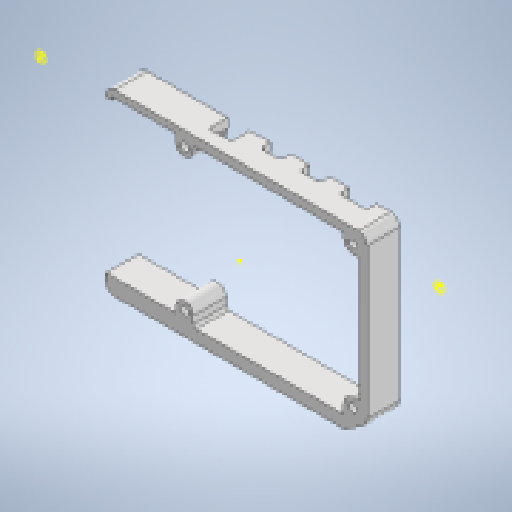
# Autodesk Inventor part: rpi_wspornik
Saved by Autodesk Inventor 2023.4 (Build 274418000, 418)
## iProperties
Created: 2024-09-15
Part Number: rpi_wspornik
Material: Generic
Document SubType Name: Modeling
Designer: komputer
Density: 1 g/cm^3
Appearance: Default
Author: komputer
Autodesk Inventor part; units mm, degrees
ref_plane "YZ Plane" through (0, 0, 0) normal (1, 0, 0) x (0, 1, 0)
ref_plane "XZ Plane" through (0, 0, 0) normal (0, 1, 0) x (-1, 0, 0)
ref_plane "XY Plane" through (0, 0, 0) normal (0, 0, 1) x (1, 0, 0)
sketch "Sketch1" plane through (0, 0, 0) normal (0, 0, 1) x (1, 0, 0)
  circle A0 centre (39, 24.5) radius 1.35 projected
  circle A1 centre (-19, 24.5) radius 1.35 projected
  circle A2 centre (-19, -24.5) radius 1.35 projected
  circle A3 centre (39, -24.5) radius 1.35 projected
  arc A4 (42.9875, 27.416) -> (40.9875, 29.416) centre (40.9875, 27.416) ccw projected
  line L0 (42.9875, 27.416) -> (42.9875, -26.5136) projected
  line L1 (-21.0125, 29.416) -> (40.9875, 29.416) projected
  arc A5 (42.0969, -28.1777) -> (42.9875, -26.5136) centre (40.9875, -26.5136) ccw projected
  line L2 (42.0969, -28.1777) -> (31.1281, -35.4903) projected
  line L3 (-29.6767, -31.7482) -> (-23.5983, -25.6698) projected
  line L4 (-23.5983, -25.6698) -> (-23.0125, -24.2556) projected
  line L5 (-23.0125, -24.2556) -> (-23.0125, 27.416) projected
  arc A6 (-21.0125, 29.416) -> (-23.0125, 27.416) centre (-21.0125, 27.416) ccw projected
  line L6 (-42.5, 25) -> (-42.5, -25) projected
  circle A7 centre (39, 24.5) radius 3
  circle A8 centre (-19, 24.5) radius 3
  circle A9 centre (39, -24.5) radius 3
  circle A10 centre (-19, -24.5) radius 3
  line L7 (36, -21.5) -> (42, -21.5)
  line L8 (42, -21.5) -> (42, -27.5)
  line L9 (42, -27.5) -> (36, -27.5)
  line L10 (36, -27.5) -> (36, -21.5)
  line L11 (36, -21.5) -> (42, -27.5) construction
  line L12 (42, -21.5) -> (36, -27.5) construction
  line L13 (36, -27.5) -> (36, -32.2423)
  line L14 (42, -21.5) -> (42.9875, -21.5)
  line L15 (42.5, -25) -> (42.5, 25) projected
  line L16 (41.5, -21.5) -> (41.5, 38.929)
  line L17 (40, 10.3) -> (39.15, 10.3) projected
  line L18 (42.9875, 11.3) -> (36.4675, 11.3)
  line L19 (40.35, 24.5) -> (42.9875, 24.5)
  line L20 (46.88, 26.416) -> (-24.7177, 26.416)
  line L21 (-16, 24.5) -> (-16, 26.416)
  line L22 (-22, 24.5) -> (-22, 26.416)
  line L23 (-22, 26.416) -> (-22, 29.1552)
  point P0 (0, 0)
  point P1 (36.6915, 26.416)
  point P2 (41.3085, 26.416)
  point P3 (41.5, 26.416)
  point P4 (41.5, 26.1583)
  point P5 (41.5, 22.8417)
  point P6 (41.5, 24.5)
  point P7 (42.5, 24.5)
  point P8 (42.5, 11.3)
  point P9 (41.5, 11.3)
  point P10 (39, -21.5)
  point P11 (36, -24.5)
  dimension "d0" = 6
  dimension "d1" = 6
  dimension "d2" = 6
  dimension "d3" = 6
  dimension "d4" = 1
  dimension "d5" = 1
  dimension "d6" = 3
  constraints: 30 end point, 8 point on line, 5 perpendicular, 4 centre point, 4 coincident, 3 horizontal, 3 parallel, 3 point on circle, 2 midpoint, 1 horizontal alignment, 1 vertical, 1 other
  measures "d0" diameter of A7
  measures "d1" diameter of A8
  measures "d2" diameter of A9
  measures "d3" diameter of A10
  measures "d4" distance between parallel lines of L15 L16
  measures "d5" distance between parallel lines of L18 L17
  measures "d6" distance between parallel lines of L1 L20
extrude "Extrusion1" add sketch "Sketch1" along normal blind 11.2 contours L0 L20 L16 A4 | L16 L20 A7 A8 L23 A6 L1 A4 | L0 L19 A7 L16 L20 | L16 A7 L20 | L0 L18 L15 L19 | L16 A7 L20 | A7 L19 L16 | L20 A7 | L0 L14 L15 L18 | L0 A5 L2 L13 L9 L8 L14 | L15 L14 L7 L16 L18 | L20 A8 L22 | L21 A8 L20 | L20 A8 | A8 L20 | L8 A9 L7 | A9 | L8 L9 A9 | L10 A9 L9 | A10 picked at (41.5914, 25.4334)
sketch "Sketch2" plane through (0, 0, 11.2) normal (0, 0, 1) x (1, 0, 0)
  line L0 (-39.5, -28) -> (39.5, -28) projected
  line L1 (36, -32.2423) -> (42.0969, -28.1777) projected
  circle A0 centre (-19, -24.5) radius 3 projected
  line L2 (36, -32.2423) -> (-22, -32.2423)
  line L3 (-22, -32.2423) -> (-22, -24.5)
  line L4 (-16, -24.5) -> (-16, -28)
  line L5 (36, -24.5) -> (36, -32.2423) projected
  point P0 (0, 0)
  point P1 (36, -28)
  constraints: 6 end point, 2 perpendicular, 2 point on circle, 1 horizontal, 1 point on line, 1 tangent
extrude "Extrusion2" add sketch "Sketch2" against normal up to surface (11.2 mm away) contours L3 A0 L4 L0 | L0 L5 L2 L3
sketch "Sketch3" plane through (0, 0, 0) normal (0, 0, -1) x (-1, 0, 0)
  line L0 (-35.77, 29.5) -> (-35.77, 28.6) projected
  line L1 (-26.83, 29.5) -> (-26.83, 28.6) projected
  line L2 (-19.75, 28.35) -> (-19.75, 29.8) projected
  line L3 (-13.25, 29.8) -> (-13.25, 28.35) projected
  line L4 (-6.25, 28.35) -> (-6.25, 29.8) projected
  line L5 (0.25, 29.8) -> (0.25, 28.35) projected
  line L6 (8, 24.9) -> (8, 27) projected
  line L7 (15, 27) -> (15, 24.9) projected
  line L8 (-35.77, 29.5) -> (-26.83, 29.5)
  line L9 (-26.83, 29.5) -> (-26.83, 26.142)
  line L10 (-26.83, 26.142) -> (-35.77, 26.142)
  line L11 (-35.77, 26.142) -> (-35.77, 29.5)
  line L12 (-19.75, 29.8) -> (-13.15, 29.8)
  line L13 (-13.15, 29.8) -> (-13.15, 26.142)
  line L14 (-13.15, 26.142) -> (-19.75, 26.142)
  line L15 (-19.75, 26.142) -> (-19.75, 29.8)
  line L16 (-6.25, 29.8) -> (0.35, 29.8)
  line L17 (0.35, 29.8) -> (0.35, 26.142)
  line L18 (0.35, 26.142) -> (-6.25, 26.142)
  line L19 (-6.25, 26.142) -> (-6.25, 29.8)
  line L20 (-26.53, 25.842) -> (-26.53, 29.8)
  line L21 (-26.53, 29.8) -> (-36.07, 29.8)
  line L22 (-36.07, 29.8) -> (-36.07, 25.842)
  line L23 (-36.07, 25.842) -> (-26.53, 25.842)
  line L24 (-20.05, 25.842) -> (-12.85, 25.842)
  line L25 (-12.85, 25.842) -> (-12.85, 30.1)
  line L26 (-12.85, 30.1) -> (-20.05, 30.1)
  line L27 (-20.05, 30.1) -> (-20.05, 25.842)
  line L28 (-6.55, 25.842) -> (0.65, 25.842)
  line L29 (0.65, 25.842) -> (0.65, 30.1)
  line L30 (0.65, 30.1) -> (-6.55, 30.1)
  line L31 (-6.55, 30.1) -> (-6.55, 25.842)
  line L32 (8, 30.3074) -> (15, 30.3074)
  line L33 (15, 30.3074) -> (15, 24.9)
  line L34 (15, 24.9) -> (8, 24.9)
  line L35 (8, 24.9) -> (8, 30.3074)
  line L36 (7.7, 24.6) -> (15.3, 24.6)
  line L37 (15.3, 24.6) -> (15.3, 30.6074)
  line L38 (15.3, 30.6074) -> (7.7, 30.6074)
  line L39 (7.7, 30.6074) -> (7.7, 24.6)
  line L40 (2.5, 26.8) -> (2.5, 23.7709) projected
  line L41 (5.5, 26.8) -> (5.5, 23.7709) projected
  line L42 (5.5, 23.7709) -> (2.5, 23.7709)
  line L43 (2.5, 23.7709) -> (2.5, 28.416)
  line L44 (2.5, 28.416) -> (5.5, 28.416)
  line L45 (5.5, 28.416) -> (5.5, 23.7709)
  line L46 (-40.9875, 29.416) -> (21.0125, 29.416) projected
  point P0 (0, 0)
  dimension "d11" = 0.3
  dimension "d12" = 0.3
  dimension "d13" = 0.3
  dimension "d14" = 0.3
  dimension "d15" = 1
  constraints: 72 end point, 18 parallel, 9 perpendicular, 5 horizontal, 2 point on line, 12 other
  measures "d11" distance between parallel lines of L9 L20
  measures "d12" distance between parallel lines of L14 L24
  measures "d13" distance between parallel lines of L18 L28
  measures "d14" distance between parallel lines of L34 L36
  measures "d15" distance between parallel lines of L44 L46
extrude "Extrusion3" cut sketch "Sketch3" against normal blind 3.5
sketch "Sketch4" plane through (0, 0, 3.5) normal (0, 0, -1) x (-1, 0, 0)
  line L0 (5.5, 26.416) -> (2.5, 26.416) projected
  line L1 (5.5, 28.416) -> (5.5, 26.416) projected
  line L2 (2.5, 28.416) -> (5.5, 28.416) projected
  line L3 (2.5, 26.416) -> (2.5, 28.416) projected
  point P0 (0, 0)
extrude "Extrusion4" cut sketch "Sketch4" against normal blind 3
sketch "Sketch5" plane through (0, 0, 3.5) normal (0, 0, -1) x (-1, 0, 0)
  line L0 (15.3, 26.416) -> (7.7, 26.416) projected
  line L1 (15.3, 29.416) -> (15.3, 26.416) projected
  line L2 (7.7, 29.416) -> (15.3, 29.416) projected
  line L3 (7.7, 26.416) -> (7.7, 29.416) projected
  point P0 (0, 0)
extrude "Extrusion5" cut sketch "Sketch5" against normal blind 3
fillet "Fillet1" radius 1 6 edges at (26.53, 27.916, 3.5) (36.07, 27.916, 3.5) (20.05, 27.916, 3.5) (12.85, 27.916, 3.5) (-0.65, 27.916, 3.5) (6.55, 27.916, 3.5)
fillet "Fillet2" radius 0.5 2 edges at (-7.7, 27.916, 6.5) (-15.3, 27.916, 6.5)
fillet "Fillet3" radius 2 2 edges at (-22, -32.2423, 5.6) (36, -32.2423, 5.6)
sketch "Sketch6" plane through (0, 0, 11.2) normal (0, 0, 1) x (1, 0, 0)
  line L0 (41.5, 24.5) -> (42.5, 24.5) projected
  line L1 (42.5, 24.5) -> (42.5, 11.3) projected
  line L2 (41.5, 22.8417) -> (41.5, 24.5) projected
  arc A0 (36.6915, 26.416) -> (41.5, 22.8417) centre (39, 24.5) ccw projected
  line L3 (42.5, 11.3) -> (41.5, 11.3) projected
  line L4 (41.5, 11.3) -> (41.5, 22.8417)
  line L5 (39, 21.5) -> (41.5, 21.5)
  line L6 (-16, 26.416) -> (36.6915, 26.416) projected
  line L7 (36, 24.5) -> (36, 26.416)
  point P0 (0, 0)
  constraints: 6 end point, 2 perpendicular, 2 point on circle, 2 point on line
extrude "Extrusion6" add sketch "Sketch6" against normal blind 9
sketch "Sketch7" plane through (36, 26.416, 2.2) normal (0, 1, 0) x (1, 0, 0)
  arc A0 (0, -0.6676) -> (0.07, -0.3) centre (-0.93, -0.3) ccw projected
  line L0 (0.07, -0.3) -> (0.07, 0) projected
  line L1 (0, 0) -> (0.07, 0) projected
  line L2 (0, -0.6676) -> (0, 0) projected
  line L3 (-0.23, 0.82) -> (-0.23, 2.85) projected
  line L4 (0.07, 0) -> (0.07, 2.2) projected
  line L5 (0, 2.2) -> (0, -9) projected
  line L6 (0.07, 2.2) -> (0, 2.2)
  point P0 (-36, 2.2)
  constraints: 2 end point, 1 horizontal
extrude "Extrusion7" cut sketch "Sketch7" against normal blind 5
fillet "Fillet4" radius 2 1 edges at (41.5, 22.8417, 1.1)
fillet "Fillet5" radius 0.3 6 edges at (36.07, 26.416, 1.1) (36.6915, 26.416, 1.1) (42.5, 24.5, 1.1) (41.5, 24.5, 1.1) (42.5, 11.3, 1.1) (41.5, 11.3, 1.1)
fillet "Fillet6" radius 1 5 edges at (36, -28, 5.6) (41.5, -21.5, 5.6) (-16, -28, 5.6) (41.5, 21.5, 6.7) (-16, 26.416, 5.6)
sketch "Sketch8" plane through (0, 0, 11.2) normal (0, 0, 1) x (1, 0, 0)
  line L0 (-46.1, -32.2423) -> (35.3944, -32.2423) projected
  line L1 (-45.3, -25.7) -> (-24.35, -25.7) projected
  line L2 (40.9875, 29.416) -> (-46.1, 29.416) projected
  line L3 (39.5, 28) -> (-39.5, 28) projected
  line L4 (-46.1, 29.416) -> (-46.1, -32.2423) projected
  line L5 (-46.1, 27) -> (-20.2305, 27)
  line L6 (-22, 29.1552) -> (-22, 24.5) projected
  line L7 (-46.1, 27) -> (-44.1, 27)
  line L8 (-44.1, 27) -> (-44.1, 26)
  line L9 (-44.1, 26) -> (-46.1, 26)
  line L10 (-46.1, 26) -> (-46.1, 27)
  line L11 (-28.94, 7.55) -> (-45.5, 7.55) projected
  line L12 (-45.5, 12.35) -> (-29.03, 12.35) projected
  line L13 (-39.5, -28) -> (39.5, -28) projected
  line L14 (-46.1, -26.7) -> (-22, -26.7)
  line L15 (-22, -24.5) -> (-22, -30.2423) projected
  arc A0 (-22, -30.2423) -> (-20, -32.2423) centre (-20, -30.2423) ccw projected
  arc A1 (-21.0125, 29.416) -> (-22, 29.1552) centre (-21.0125, 27.416) ccw projected
  point P0 (0, 0)
  point P1 (-22, 27)
  dimension "d32" = 1
  dimension "d33" = 2
  dimension "d34" = 1
  dimension "d35" = 1
  constraints: 12 end point, 3 point on line, 2 horizontal, 2 parallel, 2 perpendicular
  measures "d32" distance between parallel lines of L3 L5
  measures "d33" distance of L8.end L9.end
  measures "d34" distance of L7.end L8.end
  measures "d35" distance between parallel lines of L14 L1
extrude "Extrusion8" add sketch "Sketch8" against normal up to surface (11.2 mm away)
sketch "Sketch9" plane through (0, 0, 11.2) normal (0, 0, 1) x (1, 0, 0)
  line L0 (43.9, 29.416) -> (-46.1, 29.416) projected
  line L1 (-46.1, 29.416) -> (-46.1, -32.2423) projected
  line L2 (-46.1, -32.2423) -> (35.3944, -32.2423) projected
  arc A0 (35.3944, -32.2423) -> (36.5038, -31.9064) centre (35.3944, -30.2423) ccw projected
  line L3 (36.5038, -31.9064) -> (43.9, -26.9757) projected
  line L4 (43.9, -26.9757) -> (43.9, 29.416) projected
  line L5 (-39.5, 28.2) -> (39.5, 28.2) projected
  arc A1 (42.7, 25) -> (39.5, 28.2) centre (39.5, 25) ccw projected
  line L6 (42.7, 25) -> (42.7, -25) projected
  arc A2 (39.5, -28.2) -> (42.7, -25) centre (39.5, -25) ccw projected
  line L7 (39.5, -28.2) -> (-39.5, -28.2) projected
  arc A3 (-42.7, -25) -> (-39.5, -28.2) centre (-39.5, -25) ccw projected
  line L8 (-42.7, -25) -> (-42.7, 25) projected
  arc A4 (-39.5, 28.2) -> (-42.7, 25) centre (-39.5, 25) ccw projected
  arc A5 (35.3944, -32.2423) -> (36.5038, -31.9064) centre (35.3944, -30.2423) ccw projected
  line L9 (36.5038, -31.9064) -> (42.0969, -28.1777) projected
  arc A6 (42.0969, -28.1777) -> (42.9875, -26.5136) centre (40.9875, -26.5136) ccw projected
  line L10 (42.9875, -26.5136) -> (42.9875, 27.416) projected
  arc A7 (42.9875, 27.416) -> (40.9875, 29.416) centre (40.9875, 27.416) ccw projected
  line L11 (40.9875, 29.416) -> (-46.1, 29.416) projected
  line L12 (-46.1, 29.416) -> (-46.1, 26) projected
  line L13 (-46.1, 26) -> (-44.1, 26) projected
  line L14 (-44.1, 26) -> (-44.1, 27) projected
  line L15 (-44.1, 27) -> (-22, 27) projected
  line L16 (-22, 27) -> (-22, 24.5) projected
  arc A8 (-22, 24.5) -> (-16, 24.5) centre (-19, 24.5) ccw projected
  line L17 (-16, 24.5) -> (-16, 25.416) projected
  arc A9 (-15, 26.416) -> (-16, 25.416) centre (-15, 25.416) ccw projected
  line L18 (-15, 26.416) -> (36, 26.416) projected
  line L19 (36, 26.416) -> (36, 24.5) projected
  arc A10 (36, 24.5) -> (39, 21.5) centre (39, 24.5) ccw projected
  line L20 (39, 21.5) -> (40.5, 21.5) projected
  arc A11 (41.5, 20.5) -> (40.5, 21.5) centre (40.5, 20.5) ccw projected
  line L21 (41.5, 20.5) -> (41.5, -20.5) projected
  arc A12 (40.5, -21.5) -> (41.5, -20.5) centre (40.5, -20.5) ccw projected
  line L22 (40.5, -21.5) -> (39, -21.5) projected
  arc A13 (39, -21.5) -> (36, -24.5) centre (39, -24.5) ccw projected
  line L23 (36, -24.5) -> (36, -27) projected
  arc A14 (35, -28) -> (36, -27) centre (35, -27) ccw projected
  line L24 (35, -28) -> (-15, -28) projected
  arc A15 (-16, -27) -> (-15, -28) centre (-15, -27) ccw projected
  line L25 (-16, -27) -> (-16, -24.5) projected
  arc A16 (-16, -24.5) -> (-22, -24.5) centre (-19, -24.5) ccw projected
  line L26 (-22, -24.5) -> (-22, -26.7) projected
  line L27 (-22, -26.7) -> (-46.1, -26.7) projected
  line L28 (-46.1, -26.7) -> (-46.1, -32.2423) projected
  line L29 (-46.1, -32.2423) -> (35.3944, -32.2423) projected
  circle A17 centre (-19, 24.5) radius 1.35 projected
  circle A18 centre (39, 24.5) radius 1.35 projected
  circle A19 centre (39, -24.5) radius 1.35 projected
  circle A20 centre (-19, -24.5) radius 1.35 projected
  point P0 (0, 0)
  point P1 (40.9875, 29.416)
extrude "Extrusion9" add sketch "Sketch9" against normal up to surface (11.2 mm away) contours L4 L3 A6 L10 A7 L0
fillet "Fillet7" radius 3 4 edges at (43.9, 29.416, 5.6) (43.9, -26.9757, 5.6) (-46.1, -32.2423, 5.6) (-46.1, 29.416, 5.6)
body "Solid1"
